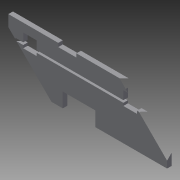
# Autodesk Inventor part: RearBulkhead
Saved by Autodesk Inventor 2014 (Build 180170000, 170)
## iProperties
Created: 2015-01-07
Part Number: RearBulkhead
Material: Generic
Document SubType Name: Modeling
Designer: Owner
Density: 1 g/cm^3
Appearance: Default
Author: Owner
Autodesk Inventor part; units mm, degrees
ref_plane "YZ Plane" through (0, 0, 0) normal (1, 0, 0) x (0, 1, 0)
ref_plane "XZ Plane" through (0, 0, 0) normal (0, 1, 0) x (-1, 0, 0)
ref_plane "XY Plane" through (0, 0, 0) normal (0, 0, 1) x (1, 0, 0)
sketch "Sketch1" plane through (0, 0, 0) normal (0, 0, 1) x (1, 0, 0)
  line L0 (117.4905, 295.341) -> (6.3655, 295.341)
  line L1 (6.3655, 295.341) -> (6.3655, 257.241)
  line L2 (6.3655, 257.241) -> (117.4905, 257.241)
  line L3 (117.4905, 257.241) -> (117.4905, 295.341)
  line L4 (117.4905, 283.403) -> (6.3655, 283.403)
  line L5 (6.3655, 283.403) -> (6.3655, 281.773)
  line L6 (6.3655, 281.773) -> (117.4905, 281.773)
  line L7 (117.4905, 281.773) -> (117.4905, 283.403)
  line L8 (117.4905, 281.773) -> (117.4905, 283.403)
  line L9 (6.3655, 283.403) -> (11.128, 283.403)
  line L10 (11.128, 283.403) -> (11.128, 281.773)
  line L11 (11.128, 281.773) -> (6.3655, 281.773)
  line L12 (6.3655, 281.773) -> (6.3655, 283.403)
  line L13 (117.4905, 283.403) -> (114.3155, 283.403)
  line L14 (114.3155, 283.403) -> (114.3155, 281.773)
  line L15 (114.3155, 281.773) -> (117.4905, 281.773)
  line L16 (117.4905, 281.773) -> (117.4905, 283.403)
  point P0 (0, 0)
  dimension "d0" = 38.1
  dimension "d1" = 111.125
  dimension "d2" = 1.63
  dimension "d3" = 11.938
  dimension "d23" = 103.1875
  dimension "d24" = 3.175
  constraints: 34 end point, 8 parallel, 6 point on line, 5 perpendicular, 4 horizontal
  measures "d0" distance of L0.end L1.end
  measures "d1" distance of L0.start L0.end
  measures "d2" distance between parallel lines of L6 L4
  measures "d3" distance between parallel lines of L0 L4
  measures "d23" distance between parallel lines of L14 L10
  measures "d24" distance between parallel lines of L3 L14
extrude "Extrusion1" add sketch "Sketch1" along normal blind 3.175 contours L3 L4 L1 L0 | L3 L6 L14 L4 | L4 L10 L6 L1 | L3 L2 L1 L6
sketch "Sketch2" plane through (0, 0, 0) normal (0, 0, -1) x (-1, 0, 0)
  line L0 (-114.3155, 283.403) -> (-11.128, 283.403) projected
  line L1 (-26.2688, 289.3188) -> (-16.7438, 289.3188)
  line L2 (-16.7438, 289.3188) -> (-16.7438, 279.7938)
  line L3 (-16.7438, 279.7938) -> (-26.2688, 279.7938)
  line L4 (-26.2688, 279.7938) -> (-26.2688, 289.3188)
  line L5 (-96.4063, 289.4015) -> (-86.8813, 289.4015)
  line L6 (-86.8813, 289.4015) -> (-86.8813, 279.8838)
  line L7 (-86.8813, 279.8838) -> (-96.4063, 279.8838)
  line L8 (-96.4063, 279.8838) -> (-96.4063, 289.4015)
  line L9 (-6.3655, 257.241) -> (-117.4905, 257.241) projected
  line L10 (-6.3655, 295.341) -> (-6.3655, 257.241) projected
  line L11 (-67.3255, 257.241) -> (-44.4655, 257.241)
  line L12 (-44.4655, 257.241) -> (-44.4655, 267.401)
  line L13 (-44.4655, 267.401) -> (-67.3255, 267.401)
  line L14 (-67.3255, 267.401) -> (-67.3255, 257.241)
  line L15 (-117.4905, 257.241) -> (-117.4905, 295.341) projected
  line L16 (-117.4905, 295.341) -> (-6.3655, 295.341) projected
  line L17 (-53.9905, 295.341) -> (-41.2905, 295.341)
  line L18 (-41.2905, 295.341) -> (-41.2905, 292.801)
  line L19 (-41.2905, 292.801) -> (-53.9905, 292.801)
  line L20 (-53.9905, 292.801) -> (-53.9905, 295.341)
  point P0 (0, 0)
  point P1 (-117.4905, 283.403)
  point P2 (-6.3655, 283.403)
  dimension "d8" = 9.525
  dimension "d9" = 9.5177
  dimension "d10" = 9.525
  dimension "d11" = 9.525
  dimension "d13" = 5.9159
  dimension "d17" = 10.16
  dimension "d18" = 22.86
  dimension "d19" = 38.1
  dimension "d20" = 2.54
  dimension "d21" = 12.7
  dimension "d22" = 63.5
  constraints: 32 end point, 8 parallel, 4 horizontal, 4 perpendicular, 2 point on line
  measures "d8" distance of L5.start L5.end
  measures "d9" distance of L5.end L6.end
  measures "d10" distance of L1.start L1.end
  measures "d11" distance of L3.end L1.start
  measures "d13" distance between parallel lines of L0 L1
  measures "d17" distance of L11.end L12.end
  measures "d18" distance of L12.end L13.end
  measures "d19" distance between parallel lines of L10 L12
  measures "d20" distance of L17.end L18.end
  measures "d21" distance of L18.end L19.end
  measures "d22" distance between parallel lines of L15 L20
extrude "Extrusion2" cut sketch "Sketch2" against normal blind 3.175 contours L8 L5 L6 L0 | L0 L6 L7 L8 | L4 L1 L2 L0 | L0 L2 L3 L4 | L9 L14 L13 L12 | L18 L19 L20 L16
body "Solid1"
